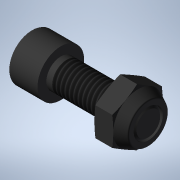
# Autodesk Inventor part: M10x30
Saved by Autodesk Inventor 2021 (Build 250183000, 183)
## iProperties
Created: 2025-06-23
Part Number: M10x30
Material: Generic
Catalog Web Link: www.cadenas.de
Description: base stand BZB-Accessories
Vendor: RNA
Document SubType Name: Modeling
Designer: psAdmin
Manufacturer: RNA
Mass: 5.61131 g
Surface Area: 24.887 cm^2
Volume: 5.61131 cm^3
Density: 1 g/cm^3
Appearance: PSOLRGB-175-175-175
Category: PARTsolutions
Company: RNA
Title: M10x30
Author: Cadenas PARTsolutions
Comments: Accessories
PSOL_IDENT_0: {$CADENAS_DATA/23d-libs/rna/bunker/zubehoer/parts/schraube_m10x30.prj},160 {VTYP=3D},{NB=M10x30},{LI
PSOL_IDENT_1: NA=M10x30},{NN=base stand BZB},{DATE=06.06.2017 07:14:33},{GEOMDATE=01.02.2017 10:28:30},{VERSION=},
PSOL_IDENT_2: {LINEID=10},{WBVAR=},{WBNUMERIC=}  {NB=M10x30},{LINA=M10x30},{KT=DUMMY},{IDNR=M10x30}
NB: M10x30
NN: base stand BZB
NT: Accessories
NBSYN: $IDNR.
LINA: M10x30
CATALOG: Rhein-Nadel-Automation
IDNR: M10x30
SUPPLIER: RNA
ARTICLENO: M10x30
BOMINFO: M10x30
CREATOR: CADENAS GmbH
Autodesk Inventor part; units mm, degrees
sketch "Sketch_1" plane through (0, 0, 0) normal (0, 0, 1) x (1, 0, 0)
  line L0 (30, 0) -> (-10, 0)
  line L1 (-10, 0) -> (-10, 7.5)
  arc A0 (-9.5, 8) -> (-10, 7.5) centre (-9.5, 7.5) ccw
  line L2 (-9.5, 8) -> (0, 8)
  line L3 (0, 8) -> (0, 5)
  line L4 (0, 5) -> (29.08, 5)
  line L5 (29.08, 5) -> (30, 4.08)
  line L6 (30, 4.08) -> (30, 0)
  line L7 (30, 0) -> (-10, 0)
  constraints: 16 end point, 2 point on circle, 1 centre point
revolve "Revolution1" add sketch "Sketch_1" angle 360 about axis through (30, 0, 0) along (1, 0, 0)
thread "Thread1" size "M10x1.5" class "6g" standard "ISO Metric profile" length 27.08
sketch "Sketch_3" plane through (-10, 0, 0) normal (-1, 0, 0) x (0, 1, 0)
  line L0 (-4, -2.3094) -> (0, -4.6188)
  line L1 (0, -4.6188) -> (4, -2.3094)
  line L2 (4, -2.3094) -> (4, 2.3094)
  line L3 (4, 2.3094) -> (0, 4.6188)
  line L4 (0, 4.6188) -> (-4, 2.3094)
  line L5 (-4, 2.3094) -> (-4, -2.3094)
  constraints: 12 end point
extrude "Extrusion1" cut sketch "Sketch_3" against normal blind 4
sketch "Sketch_4" plane through (0, 0, 0) normal (0, 0, 1) x (1, 0, 0)
  line L0 (30, 0) -> (20, 0)
  line L1 (20, 8.5) -> (20, 5)
  line L2 (20, 5) -> (30, 5)
  line L3 (30, 5) -> (30, 6.4805)
  arc A0 (30, 6.4805) -> (29.7192, 6.9299) centre (29.5, 6.4805) ccw
  line L4 (29.7192, 6.9299) -> (26.5, 8.5)
  line L5 (26.5, 8.5) -> (25.9306, 10.625)
  line L6 (25.9306, 10.625) -> (20.5694, 10.625)
  line L7 (20.5694, 10.625) -> (20, 8.5)
  constraints: 16 end point, 2 point on circle, 1 centre point
revolve "Revolution2" add sketch "Sketch_4" angle 360 about axis through (30, 0, 0) along (1, 0, 0)
sketch "Sketch_5" plane through (30, 0, 0) normal (1, 0, 0) x (0, 0, -1)
  line L0 (-17, -17) -> (17, -17)
  line L1 (17, -17) -> (17, 17)
  line L2 (17, 17) -> (-17, 17)
  line L3 (-17, 17) -> (-17, -17)
  line L4 (-8.5, -4.9075) -> (0, -9.815)
  line L5 (0, -9.815) -> (8.5, -4.9075)
  line L6 (8.5, -4.9075) -> (8.5, 4.9075)
  line L7 (8.5, 4.9075) -> (0, 9.815)
  line L8 (0, 9.815) -> (-8.5, 4.9075)
  line L9 (-8.5, 4.9075) -> (-8.5, -4.9075)
  constraints: 20 end point
extrude "Extrusion2" cut sketch "Sketch_5" against normal blind 10
ref_plane "SCHRAUBE_XY" through (0, 0, 0) normal (-1, 0, 0) x (0, 0, -1)
ref_plane "SCHRAUBE_YZ" through (0, 0, 0) normal (0, 0, -1) x (0, -1, 0)
ref_plane "SCHRAUBE_ZX" through (0, 0, 0) normal (0, -1, 0) x (-1, 0, 0)
body "Solid1"
